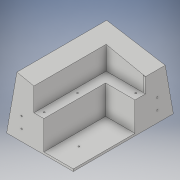
# Autodesk Inventor part: CPURightOneNew
Saved by Autodesk Inventor 2019 (Build 230136000, 136)
## iProperties
Created: 2019-01-04
Part Number: CPURightOneNew
Material: Generic
Document SubType Name: Modeling
Designer: james
Density: 1 g/cm^3
Appearance: Default
Author: james
Autodesk Inventor part; units mm, degrees
ref_plane "YZ Plane" through (0, 0, 0) normal (1, 0, 0) x (0, 1, 0)
ref_plane "XZ Plane" through (0, 0, 0) normal (0, 1, 0) x (-1, 0, 0)
ref_plane "XY Plane" through (0, 0, 0) normal (0, 0, 1) x (1, 0, 0)
sketch "Sketch1" plane through (0, 0, 0) normal (0, 1, 0) x (-1, 0, 0)
  line L0 (45.7123, 106.2129) -> (-21.5977, 106.2129)
  line L1 (-21.5977, 106.2129) -> (-21.5977, -39.8371)
  line L2 (-21.5977, -39.8371) -> (45.7123, -39.8371)
  line L3 (45.7123, -39.8371) -> (45.7123, 106.2129)
  point P0 (0, 0)
  dimension "d0" = 146.05
  dimension "d1" = 67.31
  constraints: 8 end point, 2 parallel, 1 horizontal, 1 perpendicular
  measures "d0" distance of L0.end L1.end
  measures "d1" distance of L1.end L2.end
extrude "Extrusion1" add sketch "Sketch1" along normal blind 5.08
sketch "Sketch2" plane through (21.5977, 0, 106.2129) normal (1, 0, 0) x (0, 0, -1)
  line L0 (0, 5.08) -> (146.05, 5.08) projected
  line L1 (146.05, 5.08) -> (140.97, 5.08)
  line L2 (140.97, 5.08) -> (140.97, 71.12)
  line L3 (140.97, 71.12) -> (146.05, 71.12)
  line L4 (146.05, 71.12) -> (146.05, 5.08)
  line L5 (0, 0) -> (146.05, 0) projected
  point P0 (106.2129, 0)
  dimension "d4" = 5.08
  dimension "d5" = 71.12
  constraints: 8 end point, 2 parallel, 1 horizontal, 1 perpendicular
  measures "d4" distance between parallel lines of L2 L4
  measures "d5" distance between parallel lines of L3 L5
extrude "Extrusion2" add sketch "Sketch2" against normal blind 98.425
sketch "Sketch51" plane through (-45.7123, 0, 106.2129) normal (0, 0, 1) x (1, 0, 0)
  line L0 (0, 0) -> (0, 71.12) projected
  line L1 (0, 0) -> (-5.08, 0)
  line L2 (-5.08, 0) -> (-5.08, 71.12)
  line L3 (-5.08, 71.12) -> (0, 71.12)
  line L4 (0, 71.12) -> (0, 0)
  line L5 (67.31, 71.12) -> (-31.115, 71.12) projected
  point P0 (45.7123, 0)
  dimension "d172" = 5.08
  dimension "d173" = 0
  constraints: 8 end point, 2 parallel, 1 horizontal, 1 perpendicular
  measures "d172" distance of L0.start L1.end
  measures "d173" distance between parallel lines of L3 L5
extrude "Extrusion37" add sketch "Sketch51" against normal blind 146.05
sketch "Sketch52" plane through (21.5977, 0, 106.2129) normal (1, 0, 0) x (0, 0, -1)
  line L0 (140.97, 71.12) -> (146.05, 71.12) projected
  line L1 (140.97, 5.08) -> (140.97, 71.12) projected
  line L2 (140.97, 71.12) -> (165.1, 71.12)
  line L3 (165.1, 71.12) -> (165.1, 66.04)
  line L4 (165.1, 66.04) -> (140.97, 66.04)
  line L5 (140.97, 66.04) -> (140.97, 71.12)
  point P0 (106.2129, 0)
  dimension "d176" = 5.08
  dimension "d177" = 24.13
  constraints: 8 end point, 2 parallel, 1 horizontal, 1 perpendicular
  measures "d176" distance of L2.end L3.end
  measures "d177" distance of L0.start L2.end
extrude "Extrusion38" add sketch "Sketch52" against normal blind 111.125
sketch "Sketch53" plane through (21.5977, 0, 106.2129) normal (0, 0, 1) x (1, 0, 0)
  line L0 (-67.31, 71.12) -> (-67.31, 5.08) projected
  line L1 (-72.39, 71.12) -> (-67.31, 71.12) projected
  line L2 (-67.31, 71.12) -> (-95.25, 71.12)
  line L3 (-95.25, 71.12) -> (-95.25, 66.04)
  line L4 (-95.25, 66.04) -> (-67.31, 66.04)
  line L5 (-67.31, 66.04) -> (-67.31, 71.12)
  line L6 (-98.425, 66.04) -> (-111.125, 66.04) projected
  line L7 (-111.125, 66.04) -> (-111.125, 71.12) projected
  point P0 (-21.5977, 0)
  point P1 (-125.73, 66.04)
  dimension "d180" = 0
  dimension "d255" = 27.94
  constraints: 8 end point, 2 parallel, 1 horizontal, 1 perpendicular
  measures "d180" distance between parallel lines of L4 L6
  measures "d255" distance of L0.start L2.end
extrude "Extrusion39" add sketch "Sketch53" against normal blind 165.1
sketch "Sketch55" plane through (-45.7123, 71.12, -34.7571) normal (0, 1, 0) x (1, 0, 0)
  line L0 (67.31, 0) -> (0, 0) projected
  line L1 (67.31, 0) -> (67.31, 24.13) projected
  point P0 (45.7123, -34.7571)
  point P1 (54.61, 14.605)
  dimension "d192" = 14.605
  dimension "d204" = 12.7
  measures "d192" distance from line of L0 point (54.61, 14.605)
  measures "d204" distance from line of point (54.61, 14.605) L1
hole "Hole9" at (8.8977, 71.12, -49.3621) direction (0, -1, 0) diameter 3.81 depth 25.4 tip angle 118.188
sketch "Sketch57" plane through (-45.7123, 71.12, -34.7571) normal (0, 1, 0) x (1, 0, 0)
  line L0 (0, -140.97) -> (0, 0) projected
  line L1 (0, -140.97) -> (-27.94, -140.97) projected
  point P0 (45.7123, -34.7571)
  point P1 (-12.0904, -51.8922)
  point P2 (-12.0904, -128.0922)
  dimension "d205" = 0
  dimension "d206" = 12.0904
  dimension "d207" = 76.2
  dimension "d208" = 12.8778
  measures "d205" horizontal distance of point (-12.09, -128.092) point (-12.09, -51.892)
  measures "d206" distance from line of L0 point (-12.09, -51.892)
  measures "d207" distance of point (-12.09, -128.092) point (-12.09, -51.892)
  measures "d208" distance from line of L1 point (-12.09, -128.092)
hole "Hole10" at (-57.8027, 71.12, 17.1351) at (-57.8027, 71.12, 93.3351) direction (0, -1, 0) diameter 3.302 depth 25.4 tip angle 118.188
sketch "Sketch60" plane through (21.5977, 0, 106.2129) normal (0, 0, 1) x (1, 0, 0)
  line L0 (-72.39, 0) -> (0, 0) projected
  line L1 (-147.32, 0) -> (-152.4, 0)
  line L2 (-147.32, 0) -> (-117.3637, 169.8909)
  line L3 (-98.425, 5.08) -> (-98.425, 66.04) projected
  line L4 (-152.4, 0) -> (-122.4437, 169.8909)
  line L5 (-117.3637, 169.8909) -> (-122.4437, 169.8909)
  point P0 (-21.5977, 0)
  dimension "d223" = 5.08
  dimension "d224" = 0
  dimension "d225" = 152.4
  dimension "d226" = 10
  dimension "d227" = 10
  constraints: 8 end point, 2 horizontal
  measures "d223" distance of L1.start L1.end
  measures "d224" distance between parallel lines of L0 L1
  measures "d225" distance of L0.end L1.end
  measures "d226" angle of L2 L3
  measures "d227" angle of L3 L4
extrude "Extrusion42" add sketch "Sketch60" against normal blind 228.6
sketch "Sketch66" plane through (-50.7923, 0, 106.2129) normal (0, 0, 1) x (1, 0, 0)
  line L0 (5.08, 71.12) -> (-22.86, 71.12) projected
  line L1 (-22.86, 66.04) -> (0, 66.04) projected
  line L2 (-17.78, 66.04) -> (-22.86, 66.04)
  line L3 (-22.86, 66.04) -> (-22.86, 162.1783)
  line L4 (-22.86, 162.1783) -> (-17.78, 162.1783)
  line L5 (-17.78, 162.1783) -> (-17.78, 66.04)
  line L6 (5.08, 71.12) -> (5.08, 5.08) projected
  point P0 (50.7923, 0)
  point P1 (-62.3896, 71.12)
  point P2 (-63.2854, 66.04)
  dimension "d245" = 5.08
  dimension "d252" = 22.86
  constraints: 8 end point, 2 parallel, 1 horizontal, 1 perpendicular, 1 point on line
  measures "d245" distance between parallel lines of L3 L5
  measures "d252" distance between parallel lines of L5 L6
extrude "Extrusion48" add sketch "Sketch66" against normal blind 258.445
sketch "Sketch71" plane through (21.5977, 66.04, -58.8871) normal (0, 0, -1) x (-1, 0, 0)
  line L0 (0, 5.08) -> (90.17, 5.08) projected
  line L1 (0, 5.08) -> (0, 0) projected
  line L2 (0, 5.08) -> (0, 39.2684)
  line L3 (0, 5.08) -> (153.6981, 5.08)
  line L4 (153.6981, 5.08) -> (153.6981, 71.3216)
  line L5 (0, 39.2684) -> (153.6981, 71.3216)
  point P0 (21.5977, -66.04)
  dimension "d256" = 34.1884
  dimension "d258" = 11.78
  constraints: 8 end point, 2 vertical
  measures "d256" distance of L0.start L2.end
  measures "d258" angle of L0 L5
extrude "Extrusion51" add sketch "Sketch71" along normal blind 5.08
sketch "Sketch72" plane through (21.5977, 71.12, -58.8871) normal (1, 0, 0) x (0, 0, -1)
  line L0 (0, 0) -> (5.08, 0) projected
  line L1 (0, 0) -> (0, -5.08) projected
  line L2 (-24.13, 0) -> (0, 0) projected
  line L3 (0, -5.08) -> (93.345, -5.08) projected
  line L4 (0, 0) -> (5.08, 0)
  line L5 (5.08, 0) -> (5.08, -5.08)
  line L6 (5.08, -5.08) -> (0, -5.08)
  line L7 (0, -5.08) -> (0, 0)
  point P0 (-58.8871, -71.12)
  constraints: 8 end point, 2 parallel, 1 horizontal, 1 perpendicular, 1 point on line
extrude "Extrusion52" add sketch "Sketch72" against normal blind 166.37
sketch "Sketch73" plane through (21.5977, 0, 106.2129) normal (1, 0, 0) x (0, 0, -1)
  line L0 (0, 0) -> (146.05, 0) projected
  line L1 (223.52, 0) -> (228.6, 0)
  line L2 (223.52, 0) -> (192.8198, 174.1092)
  line L3 (170.18, 105.3084) -> (170.18, 66.04) projected
  line L4 (228.6, 0) -> (197.8998, 174.1092)
  line L5 (192.8198, 174.1092) -> (197.8998, 174.1092)
  point P0 (106.2129, 0)
  dimension "d263" = 5.08
  dimension "d264" = 0
  dimension "d265" = 228.6
  dimension "d266" = 10
  dimension "d267" = 10
  constraints: 8 end point, 1 horizontal
  measures "d263" distance of L1.start L1.end
  measures "d264" distance between parallel lines of L1 L0
  measures "d265" distance of L0.start L1.end
  measures "d266" angle of L3 L2
  measures "d267" angle of L3 L4
extrude "Extrusion53" add sketch "Sketch73" against normal blind 206.0575
sketch "Sketch74" plane through (21.5977, 66.04, -58.8871) normal (0, 0, 1) x (1, 0, 0)
  line L0 (0, 39.2684) -> (-90.17, 58.073) projected
  line L1 (-90.17, 58.073) -> (0, 39.2684) projected
  line L2 (-90.17, 58.073) -> (-90.17, 52.993)
  line L3 (-90.17, 96.1383) -> (-90.17, 0) projected
  line L4 (-90.17, 52.993) -> (0, 34.1884)
  line L5 (-90.17, 58.073) -> (0, 39.2684)
  line L6 (0, 39.2684) -> (0, 34.1884)
  line L7 (0, -66.04) -> (0, 108.0692) projected
  point P0 (-21.5977, -66.04)
  dimension "d270" = 5.08
  dimension "d271" = 0
  constraints: 8 end point, 2 point on line, 1 collinear
  measures "d270" distance of L0.end L2.end
  measures "d271" angle of L4 L0
extrude "Extrusion54" add sketch "Sketch74" against normal blind 50.8
sketch "Sketch75" plane through (21.5977, 66.04, -58.8871) normal (0, 0, 1) x (1, 0, 0)
  line L0 (-95.25, 59.1325) -> (-124.1847, 65.1667) projected
  line L1 (-124.1847, 65.1667) -> (-95.25, 59.1325)
  line L2 (-95.25, 59.1325) -> (-95.25, 53.9432)
  line L3 (-95.25, 96.1383) -> (-95.25, 0) projected
  line L4 (-95.25, 53.9432) -> (-125.0673, 60.1615)
  line L5 (-124.1847, 65.1667) -> (-95.25, 59.1325) projected
  line L6 (-124.1847, 65.1667) -> (-125.0673, 60.1615)
  line L7 (-135.6754, 0) -> (-124.1847, 65.1667) projected
  point P0 (-21.5977, -66.04)
  dimension "d274" = 5.08
  constraints: 8 end point, 1 parallel, 1 point on line
  measures "d274" distance between parallel lines of L4 L0
extrude "Extrusion55" add sketch "Sketch75" against normal blind 50.8
sketch "Sketch76" plane through (-50.7923, 0, 106.2129) normal (0, 0, 1) x (1, 0, 0)
  line L0 (72.39, 105.3084) -> (-17.78, 124.113) projected
  line L1 (-22.86, 125.1725) -> (-51.7947, 131.2067) projected
  line L2 (-56.6945, 132.2285) -> (-81.3081, 137.3616) projected
  line L3 (-81.3081, 137.3616) -> (72.39, 105.3084)
  line L4 (72.39, 105.3084) -> (72.39, 181.982)
  line L5 (72.39, 181.982) -> (-81.3081, 181.982)
  line L6 (-81.3081, 137.3616) -> (-81.3081, 181.982)
  point P0 (50.7923, 0)
  constraints: 8 end point, 2 vertical, 1 perpendicular
extrude "Extrusion56" cut sketch "Sketch76" against normal blind 312.7375
sketch "Sketch77" plane through (21.5977, 66.04, -58.8871) normal (0, 0, 1) x (1, 0, 0)
  line L0 (-95.25, 59.1325) -> (-124.1847, 65.1667) projected
  line L1 (-95.25, 59.1325) -> (-95.25, 0) projected
  line L2 (-124.1847, 65.1667) -> (-147.32, -66.04) projected
  line L3 (-124.1847, 65.1667) -> (-125.0673, 60.1615) projected
  line L4 (-124.1847, 65.1667) -> (-95.25, 59.1325)
  line L5 (-129.0845, 66.1885) -> (-124.1847, 65.1667) projected
  line L6 (-124.1853, 65.1668) -> (-125.0677, 60.1615)
  line L7 (-124.1847, 65.1667) -> (-147.32, -66.04) projected
  line L8 (-95.25, 59.1325) -> (-95.25, 53.9432)
  line L9 (-125.0673, 60.1615) -> (-95.25, 53.9432) projected
  line L10 (-95.25, 53.9432) -> (-125.0677, 60.1615)
  point P0 (-21.5977, -66.04)
  constraints: 8 end point, 2 collinear, 2 point on line
extrude "Extrusion57" add sketch "Sketch77" along normal blind 165.1
sketch "Sketch78" plane through (-50.7923, 0, 106.2129) normal (0, 0, 1) x (1, 0, 0)
  line L0 (-80.01, 0) -> (-56.6945, 132.2285) projected
  line L1 (-80.01, 0) -> (-38.7202, 234.1662)
  line L2 (-38.7202, 234.1662) -> (-196.8112, 234.1662)
  line L3 (-196.8112, 234.1662) -> (-196.8112, 0)
  line L4 (-80.01, 0) -> (-196.8112, 0)
  point P0 (50.7923, 0)
  constraints: 8 end point, 2 horizontal, 1 perpendicular, 1 point on line
extrude "Extrusion58" cut sketch "Sketch78" against normal blind 303.2125
sketch "Sketch79" plane through (-76.8273, 5.08, -34.7571) normal (0, 0, 1) x (1, 0, 0)
  line L0 (3.175, 66.04) -> (-12.7, 66.04) projected
  line L1 (3.175, 60.96) -> (3.175, 66.04) projected
  line L2 (0, 60.96) -> (-12.7, 60.96) projected
  line L3 (-12.7, 60.96) -> (-12.7, 66.04) projected
  line L4 (3.175, 66.04) -> (-12.7, 66.04)
  line L5 (-12.7, 66.04) -> (-12.7, 60.96)
  line L6 (-12.7, 60.96) -> (3.175, 60.96)
  line L7 (3.175, 60.96) -> (3.175, 66.04)
  point P0 (76.8273, -5.08)
  constraints: 8 end point, 2 parallel, 1 horizontal, 1 perpendicular
extrude "Extrusion59" cut sketch "Sketch79" against normal blind 23.8125
sketch "Sketch80" plane through (21.5977, 0, 106.2129) normal (1, 0, 0) x (0, 0, -1)
  line L0 (223.52, 0) -> (228.6, 0) projected
  line L1 (228.6, 0) -> (195.4937, 187.755)
  line L2 (228.6, 0) -> (210.927, 100.2284) projected
  line L3 (195.4937, 187.755) -> (303.9198, 187.755)
  line L4 (303.9198, 187.755) -> (305.8121, 0)
  line L5 (228.6, 0) -> (305.8121, 0)
  point P0 (106.2129, 0)
  constraints: 8 end point, 2 horizontal, 1 collinear
extrude "Extrusion60" cut sketch "Sketch80" against normal blind 352.425
sketch "Sketch81" plane through (21.5977, 0, 106.2129) normal (1, 0, 0) x (0, 0, -1)
  line L0 (228.6, 0) -> (210.0313, 105.3084) projected
  line L1 (228.6, 0) -> (210.0313, 105.3084)
  line L2 (210.0313, 105.3084) -> (164.7825, 105.3084)
  line L3 (164.7825, 71.12) -> (164.7825, 66.04) projected
  line L4 (164.7825, 105.3084) -> (164.7825, 71.12)
  line L5 (140.97, 5.08) -> (140.97, 71.12) projected
  line L6 (0, 0) -> (146.05, 0) projected
  line L7 (164.7825, 71.12) -> (140.97, 71.12)
  line L8 (140.97, 71.12) -> (140.97, 0)
  line L9 (223.52, 0) -> (228.6, 0) projected
  line L10 (140.97, 0) -> (228.6, 0)
  point P0 (106.2129, 0)
  constraints: 12 end point, 3 horizontal, 2 perpendicular, 1 collinear, 1 point on line
extrude "Extrusion61" add sketch "Sketch81" against normal blind 5.08
sketch "Sketch82" plane through (-50.7923, 0, 106.2129) normal (0, 0, 1) x (1, 0, 0)
  line L0 (-80.01, 0) -> (-56.6945, 132.2285) projected
  line L1 (-17.78, 124.113) -> (-56.6945, 132.2285) projected
  line L2 (-17.78, 124.113) -> (-17.78, 71.12) projected
  line L3 (5.08, 71.12) -> (-17.78, 71.12) projected
  line L4 (5.08, 71.12) -> (5.08, 5.08) projected
  line L5 (0, 0) -> (72.39, 0) projected
  line L6 (5.08, 71.12) -> (5.08, 5.08) projected
  line L7 (5.08, 71.12) -> (5.08, 0)
  line L8 (67.31, 0) -> (0, 0) projected
  line L9 (-74.93, 0) -> (-80.01, 0) projected
  line L10 (5.08, 0) -> (-80.01, 0)
  line L11 (-80.01, 0) -> (-56.6945, 132.2285)
  line L12 (-17.78, 124.113) -> (-56.6945, 132.2285)
  line L13 (67.31, 71.12) -> (-17.78, 71.12) projected
  line L14 (-17.78, 124.113) -> (-17.78, 71.12)
  line L15 (-17.78, 71.12) -> (5.08, 71.12)
  point P0 (50.7923, 0)
  constraints: 12 end point, 4 collinear, 1 perpendicular, 1 point on line, 1 vertical
extrude "Extrusion62" add sketch "Sketch82" against normal blind 5.08
sketch "Sketch84" plane through (-114.0776, 66.04, -63.9671) normal (0, -1, 0) x (1, 0, 0)
  line L0 (40.4254, -41.6954) -> (45.5054, -41.6954) projected
  line L1 (40.4254, 0) -> (40.4254, -41.6954) projected
  line L2 (130.5954, 0) -> (130.5954, 24.13) projected
  line L3 (40.4254, 24.13) -> (130.5954, 24.13) projected
  line L4 (40.4254, 24.13) -> (40.4254, 5.3975) projected
  line L5 (40.4254, 5.3975) -> (24.5504, 5.3975) projected
  line L6 (24.5504, 5.08) -> (24.5504, 5.3975) projected
  line L7 (24.5504, 5.08) -> (0, 5.08) projected
  line L8 (0, 0) -> (0, 5.08) projected
  line L9 (40.4254, 0) -> (0, 0) projected
  line L10 (40.4254, 0) -> (40.4254, -41.6954) projected
  line L11 (40.4254, -41.6954) -> (45.5054, -41.6954) projected
  line L12 (45.5054, 0) -> (45.5054, -41.6954) projected
  line L13 (130.5954, 0) -> (45.5054, 0) projected
  circle A0 centre (122.9754, 14.605) radius 1.905 projected
  line L14 (45.5054, 0) -> (45.5054, -41.6954) projected
  line L15 (-16.7246, 170.18) -> (135.6754, 170.18) projected
  line L16 (45.5054, 5.08) -> (45.5054, 170.18) projected
  line L17 (40.4254, -41.6954) -> (45.5054, -41.6954)
  line L18 (45.5054, -41.6954) -> (45.5054, 170.18)
  line L19 (45.5054, 170.18) -> (40.4254, 170.18)
  line L20 (40.4254, 170.18) -> (40.4254, -41.6954)
  point P0 (114.0776, 63.9671)
  constraints: 8 end point, 2 parallel, 1 horizontal, 1 perpendicular
extrude "Extrusion63" add sketch "Sketch84" along normal blind 66.04 contours L1 L20 L4 L3 L16 L18 L12 L0 | L20 L15 L16 L3
sketch "Sketch85" plane through (21.5977, 5.08, -34.7571) normal (1, 0, 0) x (0, 0, -1)
  line L0 (0, 0) -> (0, 66.04) projected
  line L1 (-140.97, -5.08) -> (87.63, -5.08) projected
  point P0 (-34.7571, -5.08)
  point P1 (50.8, 20.32)
  point P2 (50.8, 45.72)
  dimension "d293" = 50.8
  dimension "d294" = 50.8
  dimension "d295" = 25.4
  dimension "d296" = 25.4
  measures "d293" distance from line of L0 point (50.8, 20.32)
  measures "d294" distance from line of L0 point (50.8, 45.72)
  measures "d295" distance from line of L1 point (50.8, 20.32)
  measures "d296" distance of point (50.8, 45.72) point (50.8, 20.32)
hole "Hole11" at (21.5977, 25.4, -85.5571) at (21.5977, 50.8, -85.5571) direction (-1, 0, 0) diameter 3.302 depth 25.4 tip angle 118.188
sketch "Sketch86" plane through (-45.7123, 5.08, 106.2129) normal (0, 0, 1) x (1, 0, 0)
  line L0 (0, 66.04) -> (0, 0) projected
  line L1 (-85.09, -5.08) -> (67.31, -5.08) projected
  point P0 (45.7123, -5.08)
  point P1 (-50.8, 20.32)
  point P2 (-50.8, 45.72)
  dimension "d304" = 50.8
  dimension "d305" = 50.8
  dimension "d306" = 25.4
  dimension "d307" = 25.4
  measures "d304" distance from line of L0 point (-50.8, 45.72)
  measures "d305" distance from line of L0 point (-50.8, 20.32)
  measures "d306" distance from line of L1 point (-50.8, 20.32)
  measures "d307" distance of point (-50.8, 45.72) point (-50.8, 20.32)
hole "Hole12" at (-96.5123, 25.4, 106.2129) at (-96.5123, 50.8, 106.2129) direction (0, 0, -1) diameter 3.302 depth 25.4 tip angle 118.188
sketch "Sketch87" plane through (-114.0776, 66.04, -63.9671) normal (0, -1, 0) x (1, 0, 0)
  line L0 (40.4254, 0) -> (0, 0) projected
  line L1 (40.4254, 5.3975) -> (24.5504, 5.3975) projected
  line L2 (130.5954, -53.34) -> (130.5954, 24.13) projected
  line L3 (130.5954, 0) -> (130.5954, 24.13) projected
  line L4 (0, 0) -> (130.5954, 0)
  line L5 (130.5954, 0) -> (130.5954, 5.3975)
  line L6 (130.5954, 5.3975) -> (0, 5.3975)
  line L7 (0, 5.3975) -> (0, 0)
  point P0 (114.0776, 63.9671)
  constraints: 8 end point, 2 parallel, 1 horizontal, 1 perpendicular, 1 point on line
extrude "Extrusion64" add sketch "Sketch87" along normal blind 66.04
sketch "Sketch88" plane through (0, 0, 0) normal (0, -1, 0) x (1, 0, 0)
  line L0 (21.5977, 106.2129) -> (21.5977, -122.3871) projected
  line L1 (-130.8023, 106.2129) -> (21.5977, 106.2129) projected
  point P0 (0, 0)
  point P1 (-16.5023, 55.4129)
  dimension "d317" = 38.1
  dimension "d318" = 50.8
  measures "d317" distance from line of L0 point (-16.502, 55.413)
  measures "d318" distance from line of L1 point (-16.502, 55.413)
hole "Hole13" at (-16.5023, 0, 55.4129) direction (0, 1, 0) diameter 3.302 depth 25.4 tip angle 118.188
equation "\"d0\" = CPDLengthHole"
equation "\"d2\" = WallWidth"
equation "\"d4\" = WallWidth"
equation "\"d5\" = CPDeckHeight"
equation "\"d172\" = WallWidth"
equation "\"d176\" = WallWidth"
equation "\"d223\" = WallWidth"
equation "\"d245\" = WallWidth"
equation "\"d259\" = WallWidth"
equation "\"d263\" = WallWidth"
equation "\"d270\" = WallWidth"
equation "\"d274\" = WallWidth"
equation "\"d287\" = WallWidth"
equation "\"d289\" = WallWidth"
equation "\"DSLength\" = 1371.6"
equation "\"DSWidth\" = 304.8"
equation "\"DCDeckHeight\" = 76.2"
equation "\"WallWidth\" = 5.08"
equation "\"EdgeAngle\" = 10deg"
equation "\"LengthCuts\" = 152.4"
equation "\"WidthCuts\" = 50.8"
equation "\"PartLength\" = 228.6"
equation "\"PartWidth\" = 152.4"
equation "\"BoltHoldDiam\" = 6.35"
equation "\"ControlPlateLength\" = 228.6"
equation "\"ControlPlateWidth\" = 228.6"
equation "\"ControlPlateShelfLength\" = 19.05"
equation "\"ControlHoleLength\" = 190.5"
equation "\"ControlHoleWidth\" = 190.5"
equation "\"ControlHoleFromSide\" = 63.5"
equation "\"ControlHoleBoltHoleMid\" = 9.525"
equation "\"CPDeckHeight\" = 71.12"
equation "\"CPFromSide\" = 63.5"
equation "\"CPFromBack\" = 63.5"
equation "\"DU1CHWidth\" = 69.85"
equation "\"DU1CHLength\" = 146.05"
equation "\"ControlPlateScrewLength\" = 76.2"
equation "\"DSBackHeight\" = 127"
equation "\"BackShelf\" = 25.4"
equation "\"MainAngle\" = 168.22deg"
equation "\"CPDWidthHole\" = 120.65"
equation "\"CPDLengthHole\" = 146.05"
equation "\"DownBackHeight\" = 130.7084"
body "Solid1"
